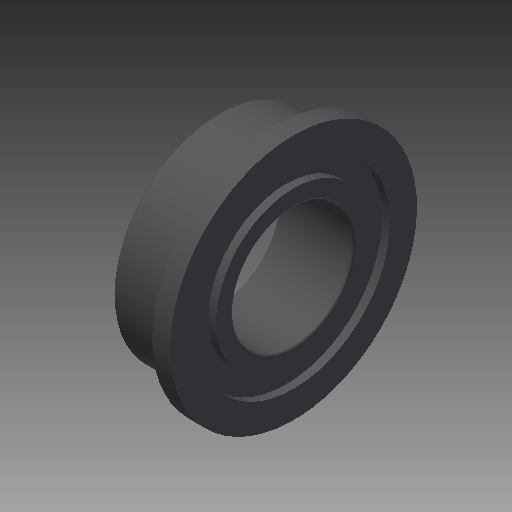
# Autodesk Inventor part: Parts_bearing_FL674ZZ
Saved by Autodesk Inventor 2018.2 (Build 222227000, 227)
## iProperties
Category: PARTsolutions
Company: MISUMI
Created: 2017-09-26
Part Number: Parts_bearing_FL674ZZ
Catalog Web Link: www.cadenas.de
Description: FL6 _ _ ZZ, FL6 _ _ AZZ, SFL6 _ _ ZZ, SFL6 _ _ AZZ, MFL1 _ _ ZZ, SMFL1 _ _ ZZ-Flanged Ball Bearings (Small Diameter, Deep Groove) - Double Shield Type
Vendor: MISUMI
Document SubType Name: Modeling
Designer: psAdmin
Manufacturer: MISUMI
Mass: 0.0672123 g
Surface Area: 1.90745 cm^2
Volume: 0.0672123 cm^3
Density: 1 g/cm^3
Material: 一般
Appearance: PSOLRGB-175-175-175
PSOL_IDENT_0: {$CADENAS_DATA\23d-libs\misumi\metric\12_bearing_holders\sfl608zz.prj},230 {VTYP=3D},{NB=FL674ZZ},{L
PSOL_IDENT_1: INA=FL674ZZ},{NN=FL6 _ _ ZZ, FL6 _ _ AZZ, SFL6 _ _ ZZ, SFL6 _ _ AZZ, MFL1 _ _ ZZ, SMFL1 _ _ ZZ},{DAT
PSOL_IDENT_2: E=16.08.2017 04:46:26},{GEOMDATE=16.08.2017 04:27:24},{VERSION=},{LINEID=40},{LINESUBID=-1},{WBVAR=M
PSOL_IDENT_3: AT}  {NB=FL674ZZ},{LINA=FL674ZZ},{KT=DUMMY},{PN=FL674ZZ},{MAT=},{MAT1= '', '52100 Bearing Steel', 'S'
PSOL_IDENT_4: , '440C Stainless Steel'},{BN=674ZZ},{DD=4.0},{AA=1.9900},{BB=0.3000},{C1=0.5750},{D=7},{B=2.5},{D1=
PSOL_IDENT_5: 8.2},{C=0.6},{RR=0.08},{CR=222},{COR=88},{CRS=222},{CRSS=217},{CORS=88},{CORSS=86},{DS=4.60},{R=0.08
PSOL_IDENT_6: },{MASS=0.35},{MAT11=1},{MMMM=}
NN: FL6 _ _ ZZ, FL6 _ _ AZZ, SFL6 _ _ ZZ, SFL6 _ _ AZZ, MFL1 _ _ ZZ, SMFL1 _ _ ZZ
NT: Flanged Ball Bearings (Small Diameter, Deep Groove) - Double Shield Type
NB: FL674ZZ
NBSYN: $PN.
LINA: FL674ZZ
PN: FL674ZZ
MAT: 52100 Bearing Steel
BN: 674ZZ
DD: 4.0
D: 7
B: 2.5
D1: 8.2
C: 0.6
RR: 0.08
CR: 222
COR: 88
DS: 4.60
R: 0.08
MASS: 0.35
SUPPLIER: MISUMI
ARTICLENO: FL674ZZ
BOMINFO: FL674ZZ
CREATOR: CADENAS GmbH
Title: Parts_bearing_FL674ZZ
Author: Cadenas PARTsolutions
Comments: Flanged Ball Bearings (Small Diameter, Deep Groove) - Double Shield Type
Autodesk Inventor part; units mm, degrees
sketch "Sketch_1" plane through (0, 0, 0) normal (0, 0, 1) x (1, 0, 0)
  line L0 (7, 0) -> (-7, 0)
  arc A0 (0, 2.08) -> (0.08, 2) centre (0.08, 2.08) ccw
  line L1 (0.08, 2) -> (2.42, 2)
  arc A1 (2.42, 2) -> (2.5, 2.08) centre (2.42, 2.08) ccw
  line L2 (2.5, 2.08) -> (2.5, 2.575)
  line L3 (2.5, 2.575) -> (2.245, 2.575)
  line L4 (2.245, 2.575) -> (2.245, 3.2)
  line L5 (2.245, 3.2) -> (2.5, 3.2)
  line L6 (2.5, 3.2) -> (2.5, 4.1)
  line L7 (2.5, 4.1) -> (1.9, 4.1)
  line L8 (1.9, 4.1) -> (1.9, 3.58)
  arc A2 (1.82, 3.5) -> (1.9, 3.58) centre (1.9, 3.5) ccw
  line L9 (1.82, 3.5) -> (0.08, 3.5)
  arc A3 (0.08, 3.5) -> (0, 3.42) centre (0.08, 3.42) ccw
  line L10 (0, 3.42) -> (0, 3.2)
  line L11 (0, 3.2) -> (0.255, 3.2)
  line L12 (0.255, 3.2) -> (0.255, 2.575)
  line L13 (0.255, 2.575) -> (0, 2.575)
  line L14 (0, 2.575) -> (0, 2.08)
  constraints: 30 end point, 8 point on circle, 4 centre point
revolve "Revolution1" add sketch "Sketch_1" angle 360 about axis through (7, 0, 0) along (1, 0, 0)
ref_plane "to_housing_XY" through (0, 0, 0) normal (1, 0, 0) x (0, 0, -1)
ref_plane "to_housing_YZ" through (0, 0, 0) normal (0, 0, -1) x (0, 1, 0)
ref_plane "to_housing_ZX" through (0, 0, 0) normal (0, 1, 0) x (1, 0, 0)
body "Solid1"
